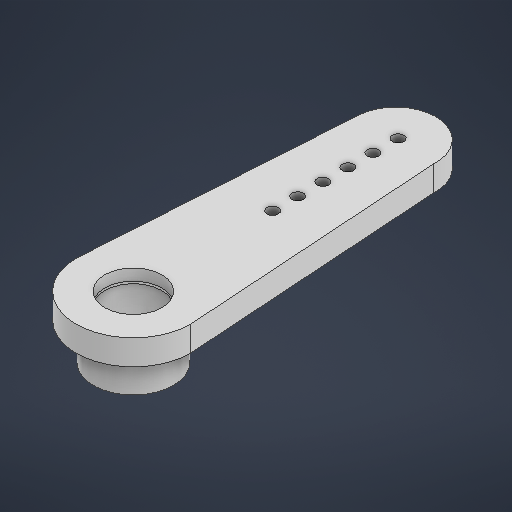
# Autodesk Inventor part: Servo Horn
Saved by Autodesk Inventor 2026.2 (Build 302298000, 298)
## iProperties
Created: 2026-03-10
Part Number: Servo Horn
Material: Generic
Document SubType Name: Modeling
Designer: chigg
Density: 1 g/cm^3
Appearance: Default
Author: chigg
Autodesk Inventor part; units mm, degrees
ref_plane "YZ Plane" through (0, 0, 0) normal (1, 0, 0) x (0, 1, 0)
ref_plane "XZ Plane" through (0, 0, 0) normal (0, 1, 0) x (-1, 0, 0)
ref_plane "XY Plane" through (0, 0, 0) normal (0, 0, 1) x (1, 0, 0)
sketch "Sketch1" plane through (0, 0, 0) normal (0, 1, 0) x (-1, 0, 0)
  arc A0 (6.3027, -103.9963) -> (-6.3005, -104.0126) centre (0, -103.172) ccw
  arc A1 (-4.4356, -132.0932) -> (4.4356, -132.6708) centre (0, -132.382) ccw
  line L0 (6.3563, -103.172) -> (4.4356, -132.6708)
  line L1 (-6.3563, -103.172) -> (-4.4356, -132.0932)
  point P0 (0, 0)
  dimension "d0" = 12.7127
  dimension "d1" = 8.89
  dimension "d2" = 29.21
  constraints: 6 point on circle, 4 end point, 2 centre point, 2 point on line, 1 tangent
  measures "d0" diameter of A0
  measures "d1" diameter of A1
  measures "d2" distance of A1.centre A0.centre
extrude "Extrusion1" add sketch "Sketch1" along normal blind 2.794 contours L0 A1 L1 A0
sketch "Sketch2" plane through (0, 0, 0) normal (0, -1, 0) x (1, 0, 0)
  circle A0 centre (0, -103.172) radius 4.445
  arc A1 (6.3563, -103.172) -> (-6.3563, -103.172) centre (0, -103.172) ccw projected
  point P0 (0, 0)
  dimension "d5" = 8.89
  dimension "d6" = 0
  constraints: 1 centre point
  measures "d5" diameter of A0
  measures "d6" distance of A1.centre A0.centre
extrude "Extrusion2" add sketch "Sketch2" along normal blind 4.064
shell "Shell1" thickness 1.27 removed faces 1 at (-0.8417, -4.064, -105.7685)
sketch "Sketch3" plane through (0, 2.794, 0) normal (0, 1, 0) x (1, 0, 0)
  circle A0 centre (0, 132.636) radius 0.635
  circle A1 centre (0, 129.842) radius 0.635
  circle A2 centre (0, 127.048) radius 0.635
  circle A3 centre (0, 124.254) radius 0.635
  circle A4 centre (0, 121.46) radius 0.635
  circle A5 centre (0, 118.666) radius 0.635
  arc A6 (4.4356, 132.0932) -> (-4.4356, 132.6708) centre (0, 132.382) ccw projected
  arc A7 (-6.3563, 103.172) -> (6.3563, 103.172) centre (0, 103.172) ccw projected
  point P0 (0, 0)
  dimension "d10" = 1.27
  dimension "d11" = 1.27
  dimension "d12" = 1.27
  dimension "d13" = 1.27
  dimension "d14" = 1.27
  dimension "d15" = 1.27
  dimension "d16" = 2.794
  dimension "d17" = 2.794
  dimension "d18" = 2.794
  dimension "d19" = 2.794
  dimension "d20" = 2.794
  dimension "d22" = 15.494
  constraints: 6 centre point
  measures "d10" diameter of A0
  measures "d11" diameter of A1
  measures "d12" diameter of A2
  measures "d13" diameter of A3
  measures "d14" diameter of A4
  measures "d15" diameter of A5
  measures "d16" distance of A4.centre A5.centre
  measures "d17" distance of A3.centre A4.centre
  measures "d18" distance of A2.centre A3.centre
  measures "d19" distance of A1.centre A2.centre
  measures "d20" distance of A0.centre A1.centre
  measures "d22" distance of A7.centre A5.centre
extrude "Extrusion3" cut sketch "Sketch3" against normal blind 4.064
sketch "Sketch4" plane through (0, 2.794, 0) normal (0, 1, 0) x (1, 0, 0)
  circle A0 centre (0, 103.172) radius 3.175 projected
  circle A1 centre (0, 103.172) radius 3.175
  point P0 (0, 0)
  constraints: 1 centre point, 1 coincident
extrude "Extrusion4" cut sketch "Sketch4" against normal blind 1.27
equation "\"d11\" = d10"
equation "\"d12\" = d11"
equation "\"d13\" = d12"
equation "\"d14\" = d10"
equation "\"d15\" = d10"
equation "\"d17\" = d16"
equation "\"d18\" = d17"
equation "\"d19\" = d18"
equation "\"d20\" = d19"
body "Solid1"
